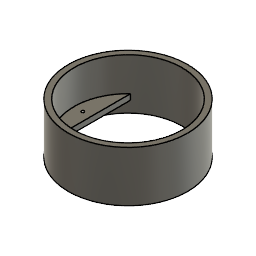
PCB CASE (Autodesk Fusion 360 design; units mm, degrees)
part number: 2026-04-27-13-45-26-943
Autodesk Fusion 360 part; units mm, degrees
sketch "Sketch1" plane through (0, 0, 0) normal (0, 1, 0) x (1, 0, 0)
  circle A0 centre (0, 0) radius 48
  circle A1 centre (0, 0) radius 53
  dimension "d1" = 96
  dimension "d2" = 106
  constraint coincident A0.centre A1.centre
  constraint concentric A0 A1
  measures "d1" diameter of A0
  measures "d2" diameter of A1
extrude "Extrude4" add sketch "Sketch1" along normal blind 10
sketch "Sketch4" plane through (0, 10, 0) normal (0, 1, 0) x (-1, 0, 0)
  circle A0 centre (0, 0) radius 48
  circle A1 centre (0, 0) radius 53
  line L0 (48, 0) -> (41.779, 0)
  line L1 (48, 0) -> (32.779, 0)
  circle A2 centre (40.279, 0) radius 1.5
  line L2 (-48, 0) -> (-32.779, 0)
  line L3 (-48, 0) -> (-41.779, 0)
  circle A3 centre (-40.279, 0) radius 1.5
  line L4 (32.779, 35.0648) -> (49, 35.0648)
  line L5 (49, 35.0648) -> (49, -35)
  line L6 (49, -35) -> (32.779, -35)
  line L7 (32.779, -35) -> (32.779, 35.0648)
  line L8 (-32.779, 35.0648) -> (-52, 35.0648)
  line L9 (-52, 35.0648) -> (-52, -35)
  line L10 (-52, -35) -> (-32.779, -35)
  line L11 (-32.779, -35) -> (-32.779, 35.0648)
  dimension "d13" = 6.221
  dimension "d14" = 15.221
  dimension "d15" = 3
  dimension "d16" = 15.221
  dimension "d17" = 6.221
  dimension "d18" = 3
  constraint coincident A0 L0.start
  constraint horizontal L0
  constraint parallel L0 L1
  constraint coincident L0.end A2
  constraint coincident A0 L2.start
  constraint horizontal L2
  constraint parallel L2 L3
  constraint coincident L3.end A3
  constraint horizontal L4
  constraint vertical L5
  constraint horizontal L6
  constraint vertical L7
  constraint coincident A0 L4.start
  constraint horizontal L8
  constraint vertical L9
  constraint horizontal L10
  constraint vertical L11
  constraint coincident A0 L8.start
  measures "d13" distance of L0.start L0.end
  measures "d14" distance of L0.start L1.end
  measures "d15" diameter of A2
  measures "d16" distance of L2.start L2.end
  measures "d17" distance of L2.start L3.end
  measures "d18" diameter of A3
extrude "Extrude5" add sketch "Sketch4" along normal blind 5 contours A0 L0 L1 A2 L7 | A0 A1 L4 L5 L6 | A0 L0 L1 A2 L6 L7 | A0 A1 L4 L8 | A0 A1 L6 L10 | A0 L2 L3 A3 L11 | A0 A1 L8 L9 L10 | A0 L2 L3 A3 L10 L11 | A1 L5 | A1 L9
sketch "Sketch5" plane through (0, 15, 0) normal (0, 1, 0) x (-1, 0, 0)
  circle A0 centre (40.279, 0) radius 1.5
  arc A1 (-32.8481, -35) -> (32.8481, -35) centre (0, 0) ccw
  line L0 (-32.8481, -35) -> (-32.779, -35)
  line L1 (-32.779, -35) -> (-32.779, 35.0648)
  arc A2 (32.779, 35.0648) -> (-32.779, 35.0648) centre (0, 0) ccw
  line L2 (32.779, 35.0648) -> (32.779, -35)
  line L3 (32.779, -35) -> (32.8481, -35)
  circle A3 centre (-40.279, 0) radius 1.5
  circle A4 centre (0, 0) radius 53
  circle A5 centre (0, 0) radius 48
  constraint coincident A1.centre A2.centre
extrude "Extrude6" add sketch "Sketch5" along normal blind 30 contours A4
thread "Thread1" "ISO Metric profile 3.0 M3x0.5 M3x0.5 6H" major diameter 3.086 minor diameter 2.529 pitch 0.5 angle 60 resizes the face on face at (-40.5395, 13.3333, -1.4772) on face at (41.1546, 13.3333, 1.2179)
